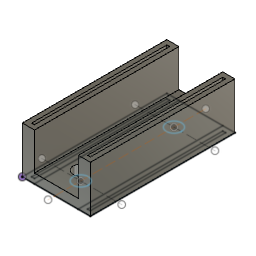
ArduinoMount (Autodesk Fusion 360 design; units mm, degrees)
Autodesk Fusion 360 part; units mm, degrees
sketch "Sketch1" plane through (0, 0, 0) normal (0, 0, 1) x (1, 0, 0)
  line L0 (0, 0) -> (18.542, 0)
  line L1 (18.542, 0) -> (18.542, 39.37)
  line L2 (18.542, 39.37) -> (0, 39.37)
  line L3 (0, 39.37) -> (0, 0)
  line L4 (3.302, 0) -> (3.302, 39.37)
  line L5 (15.24, 0) -> (15.24, 39.37)
  line L6 (16.51, 38.1) -> (17.272, 38.1)
  line L7 (17.272, 38.1) -> (17.272, 1.27)
  line L8 (17.272, 1.27) -> (16.51, 1.27)
  line L9 (16.51, 1.27) -> (16.51, 38.1)
  line L10 (1.27, 38.1) -> (2.032, 38.1)
  line L11 (2.032, 38.1) -> (2.032, 1.27)
  line L12 (2.032, 1.27) -> (1.27, 1.27)
  line L13 (1.27, 1.27) -> (1.27, 38.1)
  line L14 (-1.6611, 32.385) -> (20.0985, 32.385) construction
  line L15 (-1.6611, 6.985) -> (20.0985, 6.985) construction
  line L16 (8.9225, 41.0496) -> (8.9225, -1.9164) construction
  circle A0 centre (8.9225, 32.385) radius 2.032
  circle A1 centre (8.9225, 6.985) radius 2.032
  dimension "d1" = 18.542
  dimension "d2" = 39.37
  dimension "d3" = 3.302
  dimension "d4" = 3.302
  dimension "d5" = 36.83
  dimension "d6" = 1.27
  dimension "d7" = 0.762
  dimension "d8" = 1.27
  dimension "d9" = 36.83
  dimension "d11" = 0.762
  dimension "d12" = 1.27
  dimension "d13" = 1.27
  dimension "d26" = 6.985
  dimension "d27" = 6.985
  dimension "d28" = 4.064
  dimension "d29" = 4.064
  constraint horizontal L0
  constraint vertical L1
  constraint horizontal L2
  constraint vertical L3
  constraint coincident L0.start L3.end
  constraint coincident L0 L4.start
  constraint coincident L2 L4.end
  constraint perpendicular L2 L4
  constraint coincident L0 L5.start
  constraint coincident L2 L5.end
  constraint perpendicular L0 L5
  constraint horizontal L6
  constraint vertical L7
  constraint horizontal L8
  constraint vertical L9
  constraint horizontal L10
  constraint vertical L11
  constraint horizontal L12
  constraint vertical L13
  constraint perpendicular L1 L14
  constraint perpendicular L1 L15
  constraint perpendicular L0 L16
  constraint coincident L16 A0.centre
  constraint coincident L14 A0.centre
  constraint coincident L15 A1.centre
  constraint coincident L16 A1.centre
  measures "d1" distance of L0.start L0.end
  measures "d2" distance of L0.start L2.end
  measures "d3" distance of L1 L5
  measures "d4" distance of L3 L4
  measures "d5" distance of L6.end L7.end
  measures "d6" distance of L2 L6.start
  measures "d7" distance of L7 L9
  measures "d8" distance of L1 L7
  measures "d9" distance of L10.start L12.end
  measures "d11" distance of L11 L13
  measures "d12" distance of L3 L13
  measures "d13" distance of L2 L10.start
  measures "d26" distance of L2 L14
  measures "d27" distance of L0 L15
  measures "d28" diameter of A0
  measures "d29" diameter of A1
extrude "Extrude1" add sketch "Sketch1" along normal blind 2.54 contours L0 L2 L4 L5 | A0 | A1
extrude "Extrude2" add sketch "Sketch1" along normal blind 12.7 contours L0 L1 L2 L5
extrude "Extrude3" add sketch "Sketch1" along normal blind 12.7 contours L0 L2 L3 L4
extrude "Extrude4" add sketch "Sketch1" along normal blind 6.35 contours L6 L7 L8 L9
extrude "Extrude5" add sketch "Sketch1" along normal blind 6.35 contours L10 L11 L12 L13
extrude "Extrude6" cut sketch "Sketch1" along normal through all contours A0
extrude "Extrude7" cut sketch "Sketch1" along normal through all contours A1
